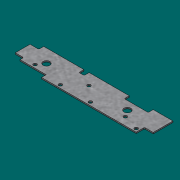
# Autodesk Inventor part: pcb_top
Saved by Autodesk Inventor 2018 (Build 220112000, 112)
## iProperties
Created: 2021-10-17
Part Number: pcb_top
Material: GFRC
Document SubType Name: Modeling
Designer: gisen
Density: 1.7 g/cm^3
Appearance: フラット - 研磨 グレー
Author: gisen
Autodesk Inventor part; units mm, degrees
ref_plane "YZ Plane" through (0, 0, 0) normal (1, 0, 0) x (0, 1, 0)
ref_plane "XZ Plane" through (0, 0, 0) normal (0, 1, 0) x (-1, 0, 0)
ref_plane "XY Plane" through (0, 0, 0) normal (0, 0, 1) x (1, 0, 0)
sketch "スケッチ1" plane through (0, 0, 0) normal (0, 0, 1) x (1, 0, 0)
  line L0 (-40.3, 9.2521) -> (-35.5, 9.2521)
  line L1 (-34.9, 9.8521) -> (-34.9, 12.3521)
  line L2 (-34.9, 12.3521) -> (-10.1, 12.3521)
  line L3 (-6.9, 12.3521) -> (17.9, 12.3521)
  line L4 (17.9, 12.3521) -> (17.9, 9.8521)
  line L5 (18.5, 9.2521) -> (32.1, 9.2521)
  line L6 (32.7, 9.8521) -> (32.7, 12.3521)
  line L7 (32.7, 12.3521) -> (44.9, 12.3521)
  line L8 (44.9, 12.3521) -> (44.9, 0.1521)
  line L9 (44.9, 0.1521) -> (40.1, 0.1521)
  line L10 (39.5, -0.4479) -> (39.5, -4.9479)
  line L11 (39.5, -4.9479) -> (-35.2, -4.9479) construction
  line L12 (-35.2, -4.9479) -> (-35.2, -2.0479) construction
  line L13 (-35.8, 0.1521) -> (-40.3, 0.1521)
  line L14 (-40.3, 0.1521) -> (-40.3, 9.2521)
  line L15 (-40.3, -0.4479) -> (-40.3, -1.5479) construction
  line L16 (-35.5, 9.3521) -> (-39.8, 9.3521) construction
  line L17 (-35, 9.8521) -> (-35, 11.8521) construction
  arc A0 (-35.5, 9.2521) -> (-34.9, 9.8521) centre (-35.5, 9.8521) ccw
  arc A1 (-35.5, 9.3521) -> (-35, 9.8521) centre (-35.5, 9.8521) ccw construction
  line L18 (-39.8, 12.3521) -> (-35.5, 12.3521) construction
  line L19 (-10, 11.8521) -> (-10, 9.8521) construction
  line L20 (-7, 9.8521) -> (-7, 11.8521) construction
  line L21 (18, 11.8521) -> (18, 9.8521) construction
  line L22 (32.6, 9.8521) -> (32.6, 11.8521) construction
  line L23 (-10.1, 12.3521) -> (-10.1, 9.8521)
  line L24 (-9.5, 9.2521) -> (-7.5, 9.2521)
  line L25 (-6.9, 9.8521) -> (-6.9, 12.3521)
  arc A2 (-10.1, 9.8521) -> (-9.5, 9.2521) centre (-9.5, 9.8521) ccw
  arc A3 (-7.5, 9.2521) -> (-6.9, 9.8521) centre (-7.5, 9.8521) ccw
  arc A4 (-10, 9.8521) -> (-9.5, 9.3521) centre (-9.5, 9.8521) ccw construction
  arc A5 (-7.5, 9.3521) -> (-7, 9.8521) centre (-7.5, 9.8521) ccw construction
  arc A6 (17.9, 9.8521) -> (18.5, 9.2521) centre (18.5, 9.8521) ccw
  arc A7 (32.1, 9.2521) -> (32.7, 9.8521) centre (32.1, 9.8521) ccw
  arc A8 (18, 9.8521) -> (18.5, 9.3521) centre (18.5, 9.8521) ccw construction
  arc A9 (32.1, 9.3521) -> (32.6, 9.8521) centre (32.1, 9.8521) ccw construction
  arc A10 (40.1, 0.0521) -> (39.6, -0.4479) centre (40.1, -0.4479) ccw construction
  arc A11 (-35.3, -0.4479) -> (-35.8, 0.0521) centre (-35.8, -0.4479) ccw construction
  arc A12 (-35.2, -0.4479) -> (-35.8, 0.1521) centre (-35.8, -0.4479) ccw
  arc A13 (40.1, 0.1521) -> (39.5, -0.4479) centre (40.1, -0.4479) ccw
  line L26 (-9.8, -5.0479) -> (-8.7, -5.0479) construction
  line L27 (45, 1.4521) -> (45, -5.1127) construction
  circle A14 centre (-25, 4.1021) radius 2.1 construction
  circle A15 centre (25, 4.1021) radius 2.1 construction
  circle A16 centre (0, 5.3521) radius 0.8 construction
  circle A17 centre (-9.25, -3.0229) radius 0.8 construction
  circle A18 centre (-27.8915, -0.0229) radius 0.8 construction
  circle A19 centre (9.25, -3.0229) radius 0.8 construction
  circle A20 centre (27.8915, -0.0229) radius 0.8 construction
  circle A21 centre (37.6, -3.0229) radius 0.8 construction
  line L28 (-17.4, 7.0521) -> (-8.6, 7.0521) construction
  line L29 (-8.6, 0.0521) -> (-17.4, 0.0521) construction
  line L30 (8.6, 7.0521) -> (17.4, 7.0521) construction
  line L31 (17.4, 0.0521) -> (8.6, 0.0521) construction
  line L32 (40.5, 7.0521) -> (32.5, 7.0521) construction
  line L33 (40.1, 0.0521) -> (32.5, 0.0521) construction
  line L34 (-39.8, 7.0521) -> (-32.5, 7.0521) construction
  line L35 (-32.5, 0.0521) -> (-35.8, 0.0521) construction
  line L36 (-13, 7.0521) -> (-13, 0.0521) construction
  line L37 (13, 7.0521) -> (13, 0.0521) construction
  line L38 (-40.3, 3.5521) -> (44.9, 3.5521) construction
  circle A22 centre (-27.8915, -0.0229) radius 1.05
  circle A23 centre (-9.25, -3.0229) radius 1.05
  circle A24 centre (9.25, -3.0229) radius 1.05
  circle A25 centre (37.6, -3.0229) radius 1.05
  circle A26 centre (25, 4.1021) radius 2.1
  circle A27 centre (-25, 4.1021) radius 2.1
  circle A28 centre (27.8915, -0.0229) radius 1.05
  circle A29 centre (0, 5.3521) radius 1.05
  circle A30 centre (-13, 3.5521) radius 2 construction
  circle A31 centre (13, 3.5521) radius 2 construction
  circle A32 centre (-37.4, 3.5521) radius 2 construction
  circle A33 centre (36.6, 3.5521) radius 2 construction
  line L39 (-26, -4.9479) -> (-26, -2.5979) construction
  line L40 (-26, -2.5979) -> (-11, -2.5979) construction
  line L41 (-11, -2.5979) -> (-11, -4.9479) construction
  arc A34 (-25.2, -2.3979) -> (-26.2, -3.3979) centre (-25.2, -3.3979) ccw construction
  arc A35 (-10.8, -3.3979) -> (-11.8, -2.3979) centre (-11.8, -3.3979) ccw construction
  line L42 (-34.8, 12.3521) -> (-34.8, 9.5521) construction
  line L43 (-34.8, 9.5521) -> (-10.2, 9.5521) construction
  line L44 (-10.2, 9.5521) -> (-10.2, 12.3521) construction
  arc A36 (-9.5, 12.3521) -> (-10, 11.8521) centre (-9.5, 11.8521) ccw construction
  arc A37 (-35, 11.8521) -> (-35.5, 12.3521) centre (-35.5, 11.8521) ccw construction
  arc A38 (-7, 11.8521) -> (-7.5, 12.3521) centre (-7.5, 11.8521) ccw construction
  arc A39 (18.5, 12.3521) -> (18, 11.8521) centre (18.5, 11.8521) ccw construction
  arc A40 (-35, 11.3521) -> (-33, 9.3521) centre (-33, 11.3521) ccw construction
  line L45 (-6.8, 12.3521) -> (-6.8, 9.5521) construction
  line L46 (-6.8, 9.5521) -> (17.8, 9.5521) construction
  line L47 (17.8, 9.5521) -> (17.8, 12.3521) construction
  line L48 (-7.5, -4.9479) -> (-7.5, -2.5979) construction
  line L49 (-7.5, -2.5979) -> (7.5, -2.5979) construction
  line L50 (7.5, -2.5979) -> (7.5, -4.9479) construction
  arc A41 (-6.7, -2.3979) -> (-7.7, -3.3979) centre (-6.7, -3.3979) ccw construction
  arc A42 (7.7, -3.3979) -> (6.7, -2.3979) centre (6.7, -3.3979) ccw construction
  line L51 (11, -4.9479) -> (11, -4.6384) construction
  line L52 (11, -4.6384) -> (11, -2.5979) construction
  line L53 (11, -2.5979) -> (26, -2.5979) construction
  line L54 (26, -2.5979) -> (26, -4.9479) construction
  arc A43 (11.8, -2.3979) -> (10.8, -3.3979) centre (11.8, -3.3979) ccw construction
  arc A44 (26.2, -3.3979) -> (25.2, -2.3979) centre (25.2, -3.3979) ccw construction
  line L55 (-35.2, -0.4479) -> (-35.2, -2.0479)
  line L56 (-35.2, -4.6657) -> (-34.5949, -4.9479) construction
  line L57 (-30.4353, -6.9979) -> (-39.7226, -2.6671) construction
  arc A45 (-19, -5.8979) -> (-21, -5.8979) centre (-20, -5.8979) ccw construction
  arc A46 (-19.4455, -4.9479) -> (-20.5545, -4.9479) centre (-20, -5.8979) ccw construction
  line L58 (-34.5949, -4.9479) -> (-20.5545, -4.9479) construction
  line L59 (-19.4455, -4.9479) -> (-19, -4.9479) construction
  line L60 (-35.2, -2.0479) -> (-19, -2.0479)
  line L61 (-19, -2.0479) -> (-19, -4.9479)
  line L62 (-39.8, -2.0479) -> (-35.8, -2.0479) construction
  line L63 (-35.2, -2.0479) -> (-35.2, -0.4479) construction
  line L64 (-19, -4.9479) -> (39.5, -4.9479)
  line L65 (-35.2, -2.0479) -> (-35.2, -4.6657) construction
  point P0 (0, 0)
  dimension "d0" = 0.1
  dimension "d3" = 0.1
  dimension "d5" = 0.1
  dimension "d8" = 0.1
  dimension "d10" = 0.1
  dimension "d11" = 0.1
  dimension "d12" = 0.1
  dimension "d13" = 2.1
  dimension "d14" = 4.2
  dimension "d15" = 24.4
  dimension "d16" = 23.6
  dimension "d17" = 4
  dimension "d18" = 0.2
  dimension "d19" = 0.2
  dimension "d20" = 0.2
  dimension "d21" = 0.2
  dimension "d22" = 0.2
  dimension "d23" = 0.2
  dimension "d24" = 0.2
  dimension "d25" = 0.2
  dimension "d26" = 0.2
  dimension "d27" = 0.2
  dimension "d28" = 0.2
  dimension "d29" = 0.2
  dimension "d30" = 0.1
  dimension "d31" = 0.1
  constraints: 90 end point, 23 perpendicular, 22 point on line, 20 centre point, 16 point on circle, 15 tangent, 13 vertical, 12 equal radius, 10 coincident, 6 concentric, 6 midpoint, 2 collinear, 2 horizontal, 1 parallel, 10 other
  measures "d0" distance between parallel lines of L16 L0
  measures "d3" distance from line of L19 L2.end
  measures "d5" distance between parallel lines of L25 L20
  measures "d8" distance between parallel lines of L21 L4
  measures "d10" distance from line of L13 L35.end
  measures "d12" distance from line of L8 L27.start
  measures "d13" diameter of A22
  measures "d14" diameter of A26
  measures "d15" distance of A30.centre A32.centre
  measures "d16" distance of A33.centre point (13, 3.552)
  measures "d17" diameter of A30
  measures "d18" distance from line of L40 A34.start
  measures "d19" distance from line of L39 A34.end
  measures "d20" distance from line of L41 A35.start
  measures "d21" distance from line of L42 L17.end
  measures "d22" distance from line of A40.end L43
  measures "d23" distance from line of L19.start L44
  measures "d24" distance from line of L45 L20.end
  measures "d25" distance from line of L21 L47.end
  measures "d26" distance from line of L48 A41.end
  measures "d27" distance from line of L50 A42.start
  measures "d28" distance from line of L52 A43.end
  measures "d29" distance from line of A44.start L54
  measures "d30" distance between parallel lines of L57 L56
  measures "d31" radial gap between concentric circles of A45 A46
extrude "押し出し1" add sketch "スケッチ1" along normal blind 0.8
equation "\"d3\" = d0"
equation "\"d5\" = d0"
equation "\"d8\" = d0"
equation "\"d10\" = d0"
equation "\"d11\" = d0"
equation "\"d12\" = d0"
equation "\"d19\" = d18"
equation "\"d20\" = d19"
equation "\"d21\" = d18"
equation "\"d22\" = d18"
equation "\"d23\" = d18"
equation "\"d24\" = d18"
equation "\"d25\" = d18"
equation "\"d26\" = d18"
equation "\"d27\" = d18"
equation "\"d28\" = d18"
equation "\"d29\" = d18"
equation "\"d30\" = d0"
equation "\"d31\" = d0"
